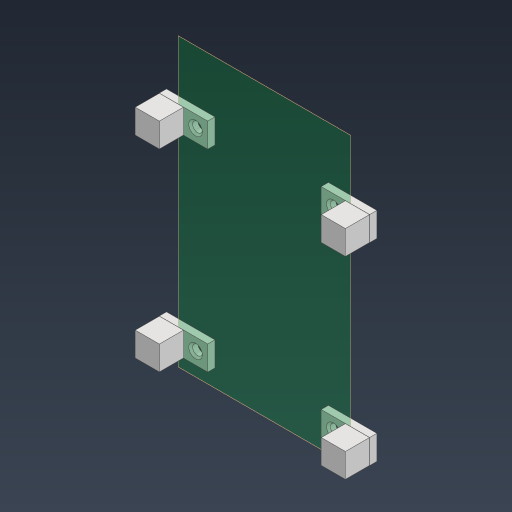
# Autodesk Inventor part: BMS_hold_check
Saved by Autodesk Inventor 2023 (Build 270158000, 158)
## iProperties
Created: 2025-12-27
Part Number: BMS_hold_check
Material: Generic
Document SubType Name: Modeling
Designer: szymo
Density: 1 g/cm^3
Appearance: Default
Author: szymo
Autodesk Inventor part; units mm, degrees
ref_plane "YZ Plane" through (0, 0, 0) normal (1, 0, 0) x (0, 1, 0)
ref_plane "XZ Plane" through (0, 0, 0) normal (0, 1, 0) x (-1, 0, 0)
ref_plane "XY Plane" through (0, 0, 0) normal (0, 0, 1) x (1, 0, 0)
ref_plane "Work Plane1" through (0, 0, -6) normal (0, 0, -1) x (-1, 0, 0)
sketch "Sketch1" plane through (0, 0, -6) normal (0, 0, -1) x (-1, 0, 0)
  circle A0 centre (-28.535, 29.86) radius 2.04 projected
  circle A1 centre (-28.535, -50.11) radius 2.04 projected
  circle A2 centre (28.535, 29.86) radius 2.04 projected
  circle A3 centre (28.535, -50.11) radius 2.04 projected
  line L0 (-30.2, -54) -> (30.2, -54) projected
  arc A4 (30.2, -54) -> (32.5, -51.7) centre (30.2, -51.7) ccw projected
  line L1 (32.5, -51.7) -> (32.5, 51.7) projected
  arc A5 (32.5, 51.7) -> (30.2, 54) centre (30.2, 51.7) ccw projected
  line L2 (30.2, 54) -> (-30.2, 54) projected
  arc A6 (-30.2, 54) -> (-32.5, 51.7) centre (-30.2, 51.7) ccw projected
  line L3 (-32.5, 51.7) -> (-32.5, -51.7) projected
  arc A7 (-32.5, -51.7) -> (-30.2, -54) centre (-30.2, -51.7) ccw projected
  line L4 (43.575, -55.15) -> (23.495, -55.15)
  line L5 (23.495, -55.15) -> (23.495, -45.07)
  line L6 (23.495, -45.07) -> (43.575, -45.07)
  line L7 (43.575, -45.07) -> (43.575, -55.15)
  line L8 (-43.575, -55.15) -> (-23.495, -55.15)
  line L9 (-23.495, -55.15) -> (-23.495, -45.07)
  line L10 (-23.495, -45.07) -> (-43.575, -45.07)
  line L11 (-43.575, -45.07) -> (-43.575, -55.15)
  line L12 (-43.575, 24.82) -> (-23.495, 24.82)
  line L13 (-23.495, 24.82) -> (-23.495, 34.9)
  line L14 (-23.495, 34.9) -> (-43.575, 34.9)
  line L15 (-43.575, 34.9) -> (-43.575, 24.82)
  line L16 (43.575, 24.82) -> (23.495, 24.82)
  line L17 (23.495, 24.82) -> (23.495, 34.9)
  line L18 (23.495, 34.9) -> (43.575, 34.9)
  line L19 (43.575, 34.9) -> (43.575, 24.82)
  circle A8 centre (28.535, -50.11) radius 5.04
  circle A9 centre (-28.535, -50.11) radius 5.04
  circle A10 centre (28.535, 29.86) radius 5.04
  circle A11 centre (-28.535, 29.86) radius 5.04
  line L20 (33.575, 34.9) -> (33.575, 24.82)
  line L21 (-33.575, 34.9) -> (-33.575, 24.82)
  line L22 (-33.575, -45.07) -> (-33.575, -55.15)
  line L23 (33.535, -45.07) -> (33.535, -55.15)
  point P0 (0, 0)
  dimension "d0" = 3
  dimension "d1" = 3
  dimension "d2" = 3
  dimension "d3" = 3
  dimension "d5" = 10
  dimension "d6" = 10
  dimension "d7" = 10
  dimension "d8" = 10
  constraints: 40 end point, 14 tangent, 8 parallel, 7 perpendicular, 7 point on line, 4 centre point, 4 horizontal, 2 midpoint
  measures "d0" radial gap between concentric circles of A3 A8
  measures "d1" radial gap between concentric circles of A1 A9
  measures "d2" radial gap between concentric circles of A2 A10
  measures "d3" radial gap between concentric circles of A0 A11
  measures "d5" distance edge to line of A8 L7
  measures "d6" distance edge to line of A9 L11
  measures "d7" distance edge to line of A11 L15
  measures "d8" distance edge to line of A10 L19
extrude "Extrusion1" add sketch "Sketch1" along normal blind 3 contours A0 | A1 | A2 | A3 | A7 L3 A9 L0 | L0 A9 L3 A7 | A9 L9 L0 | L0 L9 L8 A9 | L8 L22 A9 | A9 L10 L9 | A9 L22 L10 L3 | L3 L10 A9 | L5 A8 L0 | L0 A8 L4 L5 | L8 L11 L10 L22 | A8 L1 A4 L0 | L0 A4 L1 A8 L23 | L5 L6 A8 | L12 L21 A11 L3 | L3 A11 L12 | A8 L23 L4 | L6 L1 A8 | A11 L3 | L3 A11 | L12 L15 L14 L21 | A11 L13 L12 | L23 A8 L6 L7 L4 | L23 A8 | L6 L23 A8 L1 | A11 L21 L14 L3 | L3 L14 A11 | A11 L14 L13 | L16 A10 L1 | L1 A10 L20 L16 | A10 L1 | L1 A10 | L20 L18 L19 L16 | L16 L17 A10 | A10 L18 L1 | L1 L18 L20 A10 | L17 L18 A10
sketch "Sketch2" plane through (0, 0, -6) normal (0, 0, 1) x (1, 0, 0)
  circle A0 centre (28.535, 29.86) radius 2.04 projected
  circle A1 centre (28.535, -50.11) radius 2.04 projected
  circle A2 centre (-28.535, 29.86) radius 2.04 projected
  circle A3 centre (-28.535, -50.11) radius 2.04 projected
  line L0 (30.2, -54) -> (-30.2, -54) projected
  arc A4 (-32.5, -51.7) -> (-30.2, -54) centre (-30.2, -51.7) ccw projected
  line L1 (-32.5, -51.7) -> (-32.5, 51.7) projected
  arc A5 (-30.2, 54) -> (-32.5, 51.7) centre (-30.2, 51.7) ccw projected
  line L2 (-30.2, 54) -> (30.2, 54) projected
  arc A6 (32.5, 51.7) -> (30.2, 54) centre (30.2, 51.7) ccw projected
  line L3 (32.5, 51.7) -> (32.5, -51.7) projected
  arc A7 (30.2, -54) -> (32.5, -51.7) centre (30.2, -51.7) ccw projected
  circle A8 centre (-28.535, 29.86) radius 5
  circle A9 centre (28.535, 29.86) radius 5
  circle A10 centre (28.535, -50.11) radius 5
  circle A11 centre (-28.535, -50.11) radius 5
  line L4 (-43.535, 34.86) -> (-23.535, 34.86)
  line L5 (-23.535, 34.86) -> (-23.535, 24.86)
  line L6 (-23.535, 24.86) -> (-43.535, 24.86)
  line L7 (-43.535, 24.86) -> (-43.535, 34.86)
  line L8 (43.535, 24.86) -> (23.535, 24.86)
  line L9 (23.535, 24.86) -> (23.535, 34.86)
  line L10 (23.535, 34.86) -> (43.535, 34.86)
  line L11 (43.535, 34.86) -> (43.535, 24.86)
  line L12 (-23.535, -55.11) -> (-43.535, -55.11)
  line L13 (-43.535, -55.11) -> (-43.535, -45.11)
  line L14 (-43.535, -45.11) -> (-23.535, -45.11)
  line L15 (-23.535, -45.11) -> (-23.535, -55.11)
  line L16 (23.535, -45.11) -> (43.535, -45.11)
  line L17 (43.535, -45.11) -> (43.535, -55.11)
  line L18 (43.535, -55.11) -> (23.535, -55.11)
  line L19 (23.535, -55.11) -> (23.535, -45.11)
  line L20 (-43.575, 34.9) -> (-23.495, 34.9) projected
  line L21 (-33.535, 34.9) -> (-33.535, 24.82)
  line L22 (-23.495, 24.82) -> (-43.575, 24.82) projected
  line L23 (23.495, 34.9) -> (43.575, 34.9) projected
  line L24 (33.535, 34.9) -> (33.535, 24.86)
  line L25 (33.535, -45.11) -> (33.535, -55.11)
  line L26 (-43.575, -45.07) -> (-23.495, -45.07) projected
  line L27 (-33.535, -45.07) -> (-33.535, -55.11)
  point P0 (0, 0)
  point P1 (33.535, 34.86)
  point P2 (-33.535, 24.86)
  point P3 (-33.535, 34.86)
  point P4 (-33.535, -45.11)
  dimension "d11" = 10
  dimension "d12" = 10
  dimension "d13" = 10
  dimension "d14" = 10
  dimension "d15" = 10
  dimension "d18" = 10
  dimension "d19" = 10
  dimension "d20" = 10
  constraints: 40 end point, 16 tangent, 9 perpendicular, 8 midpoint, 8 parallel, 4 centre point, 4 coincident, 4 horizontal
  measures "d11" diameter of A8
  measures "d12" diameter of A9
  measures "d13" diameter of A10
  measures "d14" diameter of A11
  measures "d15" distance edge to line of A8 L7
  measures "d18" distance edge to line of A9 L11
  measures "d19" distance edge to line of A11 L13
  measures "d20" distance edge to line of A10 L17
extrude "Extrusion2" add sketch "Sketch2" along normal blind 10 contours L25 L16 L17 L18 | L24 L10 L11 L8 | L27 L12 L13 L14 | L6 L7 L4 L21
sketch "Sketch3" plane through (0, 0, -9) normal (0, 0, -1) x (-1, 0, 0)
  circle A0 centre (-28.535, 29.86) radius 2.04 projected
  circle A1 centre (28.535, 29.86) radius 2.04 projected
  circle A2 centre (28.535, -50.11) radius 2.04 projected
  circle A3 centre (-28.535, -50.11) radius 2.04 projected
  point P0 (0, 0)
extrude "Extrusion3" cut sketch "Sketch3" against normal through all
chamfer "Chamfer1" distance 0.8 angle 45 4 edges at (30.575, 29.86, -6) (-26.495, 29.86, -6) (-26.495, -50.11, -6) (30.575, -50.11, -6)
equation "\"d1\" = d0"
equation "\"d2\" = d0"
equation "\"d3\" = d0"
equation "\"d6\" = d5"
equation "\"d7\" = d5"
equation "\"d8\" = d5"
equation "\"d12\" = d11"
equation "\"d13\" = d11"
equation "\"d14\" = d11"
equation "\"d18\" = d15"
equation "\"d19\" = d15"
equation "\"d20\" = d15"
body "Solid1"
